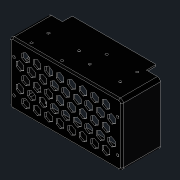
# Autodesk Inventor part: base45
Saved by Autodesk Inventor 2022 (Build 260153000, 153)
## iProperties
Created: 2021-08-30
Part Number: base45
Material: ABS プラスチック
Document SubType Name: Modeling
Designer: Yuta Kage
Density: 1.06 g/cm^3
Appearance: 滑らか - 黒
Author: Yuta Kage
Autodesk Inventor part; units mm, degrees
ref_plane "YZ Plane" through (0, 0, 0) normal (1, 0, 0) x (0, 1, 0)
ref_plane "XZ Plane" through (0, 0, 0) normal (0, 1, 0) x (-1, 0, 0)
ref_plane "XY Plane" through (0, 0, 0) normal (0, 0, 1) x (1, 0, 0)
sketch "スケッチ1" plane through (0, 0, 0) normal (0, 0, 1) x (1, 0, 0)
  line L0 (-70.25, -50) -> (70.25, -50) construction
  line L1 (70.25, -50) -> (70.25, 25) construction
  line L2 (70.25, 25) -> (-70.25, 25) construction
  line L3 (-70.25, 25) -> (-70.25, -50) construction
  line L4 (73.25, -53) -> (-73.25, -53)
  line L5 (-73.25, -53) -> (-73.25, 28)
  line L6 (-73.25, 28) -> (73.25, 28)
  line L7 (73.25, 28) -> (73.25, -53)
  point P0 (0, 0)
  dimension "d0" = 140.5
  dimension "d2" = 3
  dimension "d3" = 3
  dimension "d25" = 25
  dimension "d26" = 50
  dimension "d27" = 3
  dimension "d28" = 70.25
  dimension "d29" = 3
  constraints: 16 end point, 4 parallel, 2 horizontal, 2 perpendicular
  measures "d0" distance of L2.end L1.end
  measures "d2" distance between parallel lines of L6 L2
  measures "d3" distance between parallel lines of L5 L3
  measures "d25" distance from line of L2 point (0, 0)
  measures "d26" distance from line of L0 point (0, 0)
  measures "d27" distance between parallel lines of L1 L7
  measures "d28" distance from line of point (0, 0) L1
  measures "d29" distance between parallel lines of L0 L4
extrude "押し出し1" add sketch "スケッチ1" along normal blind 52.42
fillet "フィレット1" radius 4 4 edges at (73.25, 28, 26.21) (-73.25, 28, 26.21) (73.25, -53, 26.21) (-73.25, -53, 26.21)
fillet "フィレット2" radius 2 8 edges at (0, 28, 52.42) (-72.0784, 26.8284, 52.42) (-73.25, -12.5, 52.42) (-72.0784, -51.8284, 52.42) (0, -53, 52.42) (72.0784, -51.8284, 52.42) (73.25, -12.5, 52.42) (72.0784, 26.8284, 52.42)
shell "シェル1" thickness 2 removed faces 0
sketch "スケッチ2" plane through (0, 0, 0) normal (0, 0, -1) x (-1, 0, 0)
  arc A0 (69.25, -53) -> (73.25, -49) centre (69.25, -49) ccw projected
  line L0 (73.25, 24) -> (73.25, -49) projected
  arc A1 (73.25, 24) -> (69.25, 28) centre (69.25, 24) ccw projected
  line L1 (-69.25, 28) -> (69.25, 28) projected
  arc A2 (-69.25, 28) -> (-73.25, 24) centre (-69.25, 24) ccw projected
  line L2 (-73.25, -49) -> (-73.25, 24) projected
  arc A3 (-73.25, -49) -> (-69.25, -53) centre (-69.25, -49) ccw projected
  line L3 (69.25, -53) -> (-69.25, -53) projected
  point P0 (0, 0)
extrude "押し出し2" cut sketch "スケッチ2" against normal blind 2
sketch "スケッチ4" plane through (-69.25, -53, 50.42) normal (0, -1, 0) x (1, 0, 0)
  line L0 (138.5, -48.42) -> (0, -48.42) projected
  line L1 (124.25, -23.42) -> (14.25, -23.42)
  line L2 (14.25, -23.42) -> (14.25, -48.42)
  line L3 (14.25, -48.42) -> (124.25, -48.42)
  line L4 (124.25, -48.42) -> (124.25, -23.42)
  line L5 (124.25, -23.42) -> (14.25, -48.42) construction
  line L6 (14.25, -23.42) -> (124.25, -48.42) construction
  point P0 (69.25, -50.42)
  point P1 (69.25, -35.92)
  point P2 (69.25, -35.92)
  point P3 (124.25, -48.42)
  dimension "d21" = 110
  dimension "d22" = 25
  constraints: 12 end point, 3 midpoint, 2 parallel, 1 horizontal, 1 perpendicular, 1 point on line, 1 vertical alignment
  measures "d21" distance of L1.start L1.end
  measures "d22" distance of L3.end L1.start
extrude "押し出し3" cut sketch "スケッチ4" against normal blind 5
fillet "フィレット3" radius 5 2 edges at (55, -52, 27) (-55, -52, 27)
sketch "スケッチ3" plane through (0, 0, 52.42) normal (0, 0, 1) x (1, 0, 0)
  line L0 (73.25, 28) -> (-73.25, 28) projected
  line L1 (-73.25, 28) -> (-73.25, -53) projected
  line L2 (-73.25, -53) -> (73.25, -53) projected
  line L3 (73.25, -53) -> (73.25, 28) projected
  line L4 (-67.75, -36.75) -> (67.75, -36.75)
  line L5 (67.75, -36.75) -> (67.75, 6.75)
  line L6 (67.75, 6.75) -> (-67.75, 6.75)
  line L7 (-67.75, 6.75) -> (-67.75, -36.75)
  line L8 (-67.75, -36.75) -> (67.75, 6.75) construction
  line L9 (67.75, -36.75) -> (-67.75, 6.75) construction
  point P0 (88.6427, 28.7758)
  point P1 (88.6427, -28.7758)
  point P2 (0, 0)
  point P3 (0, -15)
  dimension "d19" = 135.5
  dimension "d20" = 43.5
  dimension "d103" = 81
  dimension "d106" = 15
  constraints: 12 end point, 2 parallel, 1 horizontal, 1 midpoint, 1 perpendicular, 1 vertical alignment
  measures "d19" distance of L5.end L6.end
  measures "d20" distance of L6.end L4.start
  measures "d103" distance between parallel lines of L2 L0
  measures "d106" distance of point (0, -15) point (0, 0)
hole "穴1" at (88.6427, -28.7758, 52.42) at (88.6427, 28.7758, 52.42) at (-67.75, 6.75, 52.42) at (-67.75, -36.75, 52.42) at (67.75, 6.75, 52.42) at (67.75, -36.75, 52.42) direction (0, 0, -1) diameter 3.4 end through all clearance for "Socket Head Cap Screw" size "M3" standard "Ansi Metric M Profile"
sketch "スケッチ5" plane through (-73.25, -49, 50.42) normal (-1, 0, 0) x (0, 0, 1)
  line L0 (-13.92, 52) -> (-21.92, 52)
  line L1 (-21.92, 52) -> (-21.92, 40)
  line L2 (-21.92, 40) -> (-13.92, 40)
  line L3 (-13.92, 40) -> (-13.92, 52)
  line L4 (-13.92, 52) -> (-21.92, 40) construction
  line L5 (-21.92, 52) -> (-13.92, 40) construction
  line L6 (0, 77) -> (-48.42, 77) projected
  line L7 (-48.42, 73) -> (-48.42, 0) projected
  line L8 (-30.92, 52) -> (-38.92, 52)
  line L9 (-38.92, 52) -> (-38.92, 40)
  line L10 (-38.92, 40) -> (-30.92, 40)
  line L11 (-30.92, 40) -> (-30.92, 52)
  line L12 (-30.92, 52) -> (-38.92, 40) construction
  line L13 (-38.92, 52) -> (-30.92, 40) construction
  point P0 (-50.42, 49)
  point P1 (-17.92, 46)
  point P2 (-34.92, 46)
  dimension "d31" = 31
  dimension "d32" = 30.5
  dimension "d33" = 8
  dimension "d34" = 12
  dimension "d37" = 17
  constraints: 24 end point, 4 midpoint, 2 horizontal, 2 parallel, 1 collinear, 1 perpendicular, 10 other
  measures "d31" distance from line of L6 point (-17.92, 46)
  measures "d32" distance from line of L7 point (-17.92, 46)
  measures "d33" distance of L1.end L2.end
  measures "d34" distance of L2.end L0.start
  measures "d37" distance of L0.start L8.start
extrude "押し出し4" cut sketch "スケッチ5" against normal blind 10
fillet "フィレット4" radius 1 8 edges at (-72.25, -9, 19.5) (-72.25, -9, 11.5) (-72.25, 3, 11.5) (-72.25, 3, 19.5) (-72.25, -9, 36.5) (-72.25, -9, 28.5) (-72.25, 3, 28.5) (-72.25, 3, 36.5)
sketch "スケッチ6" plane through (0, 0, 2) normal (0, 0, -1) x (-1, 0, 0)
  line L0 (69.25, 26) -> (-69.25, 26) projected
  line L1 (-69.25, 28) -> (69.25, 28) projected
  line L2 (55, 26) -> (-55, 26)
  line L3 (-55, 26) -> (-55, 28)
  line L4 (-55, 28) -> (55, 28)
  line L5 (55, 28) -> (55, 26)
  point P0 (0, 0)
  dimension "d45" = 55
  dimension "d46" = 55
  constraints: 8 end point, 2 parallel, 2 point on line, 1 horizontal, 1 perpendicular
  measures "d45" distance from line of point (0, 0) L3
  measures "d46" distance from line of L5 point (0, 0)
extrude "押し出し5" add sketch "スケッチ6" along normal blind 13
sketch "スケッチ7" plane through (0, 0, 52.42) normal (0, 0, 1) x (1, 0, 0)
  line L0 (-102.55, 0) -> (102.55, 0) construction
  line L1 (0, -69.2) -> (0, 44.2) projected
  line L2 (-69.25, -53) -> (69.25, -53) construction
  line L3 (69.25, 28) -> (-69.25, 28) projected
  line L4 (-60, -57.2446) -> (-65, -54.3579) construction
  line L5 (-65, -54.3579) -> (-65, -48.5844) construction
  line L6 (-65, -48.5844) -> (-60, -45.6976) construction
  line L7 (-60, -45.6976) -> (-55, -48.5844) construction
  line L8 (-55, -48.5844) -> (-55, -54.3579) construction
  line L9 (-55, -54.3579) -> (-60, -57.2446) construction
  line L10 (-67.5, -44.2543) -> (-72.5, -41.3675) construction
  line L11 (-72.5, -41.3675) -> (-72.5, -35.594) construction
  line L12 (-72.5, -35.594) -> (-67.5, -32.7073) construction
  line L13 (-67.5, -32.7073) -> (-62.5, -35.594) construction
  line L14 (-62.5, -35.594) -> (-62.5, -41.3675) construction
  line L15 (-62.5, -41.3675) -> (-67.5, -44.2543) construction
  line L16 (-60, -51.4711) -> (-67.5, -38.4808) construction
  line L17 (-57.5, -41.3675) -> (-57.5, -35.594)
  line L18 (-52.5, -44.2543) -> (-57.5, -41.3675)
  line L19 (-57.5, -35.594) -> (-52.5, -32.7073)
  line L20 (-47.5, -41.3675) -> (-52.5, -44.2543)
  line L21 (-52.5, -32.7073) -> (-47.5, -35.594)
  line L22 (-47.5, -35.594) -> (-47.5, -41.3675)
  line L23 (-50, -54.3579) -> (-50, -48.5844) construction
  line L24 (-45, -57.2446) -> (-50, -54.3579) construction
  line L25 (-50, -48.5844) -> (-45, -45.6976) construction
  line L26 (-45, -51.4711) -> (-52.5, -38.4808) construction
  line L27 (-40, -54.3579) -> (-45, -57.2446) construction
  line L28 (-40, -48.5844) -> (-40, -54.3579) construction
  line L29 (-45, -45.6976) -> (-40, -48.5844) construction
  line L30 (-72.5, -15.3868) -> (-72.5, -9.6132) construction
  line L31 (-67.5, -18.2735) -> (-72.5, -15.3868) construction
  line L32 (-72.5, -9.6132) -> (-67.5, -6.7265) construction
  line L33 (-62.5, -15.3868) -> (-67.5, -18.2735) construction
  line L34 (-67.5, -6.7265) -> (-62.5, -9.6132) construction
  line L35 (-62.5, -9.6132) -> (-62.5, -15.3868) construction
  line L36 (-65, -28.3771) -> (-65, -22.6036)
  line L37 (-60, -31.2639) -> (-65, -28.3771)
  line L38 (-65, -22.6036) -> (-60, -19.7169)
  line L39 (-60, -25.4904) -> (-67.5, -12.5) construction
  line L40 (-55, -28.3771) -> (-60, -31.2639)
  line L41 (-55, -22.6036) -> (-55, -28.3771)
  line L42 (-60, -19.7169) -> (-55, -22.6036)
  line L43 (-57.5, -15.3868) -> (-57.5, -9.6132)
  line L44 (-52.5, -18.2735) -> (-57.5, -15.3868)
  line L45 (-57.5, -9.6132) -> (-52.5, -6.7265)
  line L46 (-47.5, -15.3868) -> (-52.5, -18.2735)
  line L47 (-52.5, -6.7265) -> (-47.5, -9.6132)
  line L48 (-47.5, -9.6132) -> (-47.5, -15.3868)
  line L49 (-50, -28.3771) -> (-50, -22.6036)
  line L50 (-45, -31.2639) -> (-50, -28.3771)
  line L51 (-50, -22.6036) -> (-45, -19.7169)
  line L52 (-45, -25.4904) -> (-52.5, -12.5) construction
  line L53 (-40, -28.3771) -> (-45, -31.2639)
  line L54 (-40, -22.6036) -> (-40, -28.3771)
  line L55 (-45, -19.7169) -> (-40, -22.6036)
  line L56 (-42.5, -41.3675) -> (-42.5, -35.594)
  line L57 (-37.5, -44.2543) -> (-42.5, -41.3675)
  line L58 (-42.5, -35.594) -> (-37.5, -32.7073)
  line L59 (-32.5, -41.3675) -> (-37.5, -44.2543)
  line L60 (-37.5, -32.7073) -> (-32.5, -35.594)
  line L61 (-32.5, -35.594) -> (-32.5, -41.3675)
  line L62 (-35, -54.3579) -> (-35, -48.5844) construction
  line L63 (-30, -57.2446) -> (-35, -54.3579) construction
  line L64 (-35, -48.5844) -> (-30, -45.6976) construction
  line L65 (-30, -51.4711) -> (-37.5, -38.4808) construction
  line L66 (-25, -54.3579) -> (-30, -57.2446) construction
  line L67 (-25, -48.5844) -> (-25, -54.3579) construction
  line L68 (-30, -45.6976) -> (-25, -48.5844) construction
  line L69 (-42.5, -15.3868) -> (-42.5, -9.6132)
  line L70 (-37.5, -18.2735) -> (-42.5, -15.3868)
  line L71 (-42.5, -9.6132) -> (-37.5, -6.7265)
  line L72 (-32.5, -15.3868) -> (-37.5, -18.2735)
  line L73 (-37.5, -6.7265) -> (-32.5, -9.6132)
  line L74 (-32.5, -9.6132) -> (-32.5, -15.3868)
  line L75 (-35, -28.3771) -> (-35, -22.6036)
  line L76 (-30, -31.2639) -> (-35, -28.3771)
  line L77 (-35, -22.6036) -> (-30, -19.7169)
  line L78 (-30, -25.4904) -> (-37.5, -12.5) construction
  line L79 (-25, -28.3771) -> (-30, -31.2639)
  line L80 (-25, -22.6036) -> (-25, -28.3771)
  line L81 (-30, -19.7169) -> (-25, -22.6036)
  line L82 (-27.5, -41.3675) -> (-27.5, -35.594)
  line L83 (-22.5, -44.2543) -> (-27.5, -41.3675)
  line L84 (-27.5, -35.594) -> (-22.5, -32.7073)
  line L85 (-17.5, -41.3675) -> (-22.5, -44.2543)
  line L86 (-22.5, -32.7073) -> (-17.5, -35.594)
  line L87 (-17.5, -35.594) -> (-17.5, -41.3675)
  line L88 (-20, -54.3579) -> (-20, -48.5844) construction
  line L89 (-15, -57.2446) -> (-20, -54.3579) construction
  line L90 (-20, -48.5844) -> (-15, -45.6976) construction
  line L91 (-15, -51.4711) -> (-22.5, -38.4808) construction
  line L92 (-10, -54.3579) -> (-15, -57.2446) construction
  line L93 (-10, -48.5844) -> (-10, -54.3579) construction
  line L94 (-15, -45.6976) -> (-10, -48.5844) construction
  line L95 (-27.5, -15.3868) -> (-27.5, -9.6132)
  line L96 (-22.5, -18.2735) -> (-27.5, -15.3868)
  line L97 (-27.5, -9.6132) -> (-22.5, -6.7265)
  line L98 (-17.5, -15.3868) -> (-22.5, -18.2735)
  line L99 (-22.5, -6.7265) -> (-17.5, -9.6132)
  line L100 (-17.5, -9.6132) -> (-17.5, -15.3868)
  line L101 (-20, -28.3771) -> (-20, -22.6036)
  line L102 (-15, -31.2639) -> (-20, -28.3771)
  line L103 (-20, -22.6036) -> (-15, -19.7169)
  line L104 (-15, -25.4904) -> (-22.5, -12.5) construction
  line L105 (-10, -28.3771) -> (-15, -31.2639)
  line L106 (-10, -22.6036) -> (-10, -28.3771)
  line L107 (-15, -19.7169) -> (-10, -22.6036)
  line L108 (-12.5, -41.3675) -> (-12.5, -35.594)
  line L109 (-7.5, -44.2543) -> (-12.5, -41.3675)
  line L110 (-12.5, -35.594) -> (-7.5, -32.7073)
  line L111 (-2.5, -41.3675) -> (-7.5, -44.2543)
  line L112 (-7.5, -32.7073) -> (-2.5, -35.594)
  line L113 (-2.5, -35.594) -> (-2.5, -41.3675)
  line L114 (-5, -54.3579) -> (-5, -48.5844) construction
  line L115 (0, -57.2446) -> (-5, -54.3579) construction
  line L116 (-5, -48.5844) -> (0, -45.6976) construction
  line L117 (0, -51.4711) -> (-7.5, -38.4808) construction
  line L118 (5, -54.3579) -> (0, -57.2446) construction
  line L119 (5, -48.5844) -> (5, -54.3579) construction
  line L120 (0, -45.6976) -> (5, -48.5844) construction
  line L121 (-12.5, -15.3868) -> (-12.5, -9.6132)
  line L122 (-7.5, -18.2735) -> (-12.5, -15.3868)
  line L123 (-12.5, -9.6132) -> (-7.5, -6.7265)
  line L124 (-2.5, -15.3868) -> (-7.5, -18.2735)
  line L125 (-7.5, -6.7265) -> (-2.5, -9.6132)
  line L126 (-2.5, -9.6132) -> (-2.5, -15.3868)
  line L127 (-5, -28.3771) -> (-5, -22.6036)
  line L128 (0, -31.2639) -> (-5, -28.3771)
  line L129 (-5, -22.6036) -> (0, -19.7169)
  line L130 (0, -25.4904) -> (-7.5, -12.5) construction
  line L131 (5, -28.3771) -> (0, -31.2639)
  line L132 (5, -22.6036) -> (5, -28.3771)
  line L133 (0, -19.7169) -> (5, -22.6036)
  line L134 (2.5, -41.3675) -> (2.5, -35.594)
  line L135 (7.5, -44.2543) -> (2.5, -41.3675)
  line L136 (2.5, -35.594) -> (7.5, -32.7073)
  line L137 (12.5, -41.3675) -> (7.5, -44.2543)
  line L138 (7.5, -32.7073) -> (12.5, -35.594)
  line L139 (12.5, -35.594) -> (12.5, -41.3675)
  line L140 (10, -54.3579) -> (10, -48.5844) construction
  line L141 (15, -57.2446) -> (10, -54.3579) construction
  line L142 (10, -48.5844) -> (15, -45.6976) construction
  line L143 (15, -51.4711) -> (7.5, -38.4808) construction
  line L144 (20, -54.3579) -> (15, -57.2446) construction
  line L145 (20, -48.5844) -> (20, -54.3579) construction
  line L146 (15, -45.6976) -> (20, -48.5844) construction
  line L147 (2.5, -15.3868) -> (2.5, -9.6132)
  line L148 (7.5, -18.2735) -> (2.5, -15.3868)
  line L149 (2.5, -9.6132) -> (7.5, -6.7265)
  line L150 (12.5, -15.3868) -> (7.5, -18.2735)
  line L151 (7.5, -6.7265) -> (12.5, -9.6132)
  line L152 (12.5, -9.6132) -> (12.5, -15.3868)
  line L153 (10, -28.3771) -> (10, -22.6036)
  line L154 (15, -31.2639) -> (10, -28.3771)
  line L155 (10, -22.6036) -> (15, -19.7169)
  line L156 (15, -25.4904) -> (7.5, -12.5) construction
  line L157 (20, -28.3771) -> (15, -31.2639)
  line L158 (20, -22.6036) -> (20, -28.3771)
  line L159 (15, -19.7169) -> (20, -22.6036)
  line L160 (17.5, -41.3675) -> (17.5, -35.594)
  line L161 (22.5, -44.2543) -> (17.5, -41.3675)
  line L162 (17.5, -35.594) -> (22.5, -32.7073)
  line L163 (27.5, -41.3675) -> (22.5, -44.2543)
  line L164 (22.5, -32.7073) -> (27.5, -35.594)
  line L165 (27.5, -35.594) -> (27.5, -41.3675)
  line L166 (25, -54.3579) -> (25, -48.5844) construction
  line L167 (30, -57.2446) -> (25, -54.3579) construction
  line L168 (25, -48.5844) -> (30, -45.6976) construction
  line L169 (30, -51.4711) -> (22.5, -38.4808) construction
  line L170 (35, -54.3579) -> (30, -57.2446) construction
  line L171 (35, -48.5844) -> (35, -54.3579) construction
  line L172 (30, -45.6976) -> (35, -48.5844) construction
  line L173 (17.5, -15.3868) -> (17.5, -9.6132)
  line L174 (22.5, -18.2735) -> (17.5, -15.3868)
  line L175 (17.5, -9.6132) -> (22.5, -6.7265)
  line L176 (27.5, -15.3868) -> (22.5, -18.2735)
  line L177 (22.5, -6.7265) -> (27.5, -9.6132)
  line L178 (27.5, -9.6132) -> (27.5, -15.3868)
  line L179 (25, -28.3771) -> (25, -22.6036)
  line L180 (30, -31.2639) -> (25, -28.3771)
  line L181 (25, -22.6036) -> (30, -19.7169)
  line L182 (30, -25.4904) -> (22.5, -12.5) construction
  line L183 (35, -28.3771) -> (30, -31.2639)
  line L184 (35, -22.6036) -> (35, -28.3771)
  line L185 (30, -19.7169) -> (35, -22.6036)
  line L186 (32.5, -41.3675) -> (32.5, -35.594)
  line L187 (37.5, -44.2543) -> (32.5, -41.3675)
  line L188 (32.5, -35.594) -> (37.5, -32.7073)
  line L189 (42.5, -41.3675) -> (37.5, -44.2543)
  line L190 (37.5, -32.7073) -> (42.5, -35.594)
  line L191 (42.5, -35.594) -> (42.5, -41.3675)
  line L192 (40, -54.3579) -> (40, -48.5844) construction
  line L193 (45, -57.2446) -> (40, -54.3579) construction
  line L194 (40, -48.5844) -> (45, -45.6976) construction
  line L195 (45, -51.4711) -> (37.5, -38.4808) construction
  line L196 (50, -54.3579) -> (45, -57.2446) construction
  line L197 (50, -48.5844) -> (50, -54.3579) construction
  line L198 (45, -45.6976) -> (50, -48.5844) construction
  line L199 (32.5, -15.3868) -> (32.5, -9.6132)
  line L200 (37.5, -18.2735) -> (32.5, -15.3868)
  line L201 (32.5, -9.6132) -> (37.5, -6.7265)
  line L202 (42.5, -15.3868) -> (37.5, -18.2735)
  line L203 (37.5, -6.7265) -> (42.5, -9.6132)
  line L204 (42.5, -9.6132) -> (42.5, -15.3868)
  line L205 (40, -28.3771) -> (40, -22.6036)
  line L206 (45, -31.2639) -> (40, -28.3771)
  line L207 (40, -22.6036) -> (45, -19.7169)
  line L208 (45, -25.4904) -> (37.5, -12.5) construction
  line L209 (50, -28.3771) -> (45, -31.2639)
  line L210 (50, -22.6036) -> (50, -28.3771)
  line L211 (45, -19.7169) -> (50, -22.6036)
  line L212 (47.5, -41.3675) -> (47.5, -35.594)
  line L213 (52.5, -44.2543) -> (47.5, -41.3675)
  line L214 (47.5, -35.594) -> (52.5, -32.7073)
  line L215 (57.5, -41.3675) -> (52.5, -44.2543)
  line L216 (52.5, -32.7073) -> (57.5, -35.594)
  line L217 (57.5, -35.594) -> (57.5, -41.3675)
  line L218 (55, -54.3579) -> (55, -48.5844) construction
  line L219 (60, -57.2446) -> (55, -54.3579) construction
  line L220 (55, -48.5844) -> (60, -45.6976) construction
  line L221 (60, -51.4711) -> (52.5, -38.4808) construction
  line L222 (65, -54.3579) -> (60, -57.2446) construction
  line L223 (65, -48.5844) -> (65, -54.3579) construction
  line L224 (60, -45.6976) -> (65, -48.5844) construction
  line L225 (47.5, -15.3868) -> (47.5, -9.6132)
  line L226 (52.5, -18.2735) -> (47.5, -15.3868)
  line L227 (47.5, -9.6132) -> (52.5, -6.7265)
  line L228 (57.5, -15.3868) -> (52.5, -18.2735)
  line L229 (52.5, -6.7265) -> (57.5, -9.6132)
  line L230 (57.5, -9.6132) -> (57.5, -15.3868)
  line L231 (55, -28.3771) -> (55, -22.6036)
  line L232 (60, -31.2639) -> (55, -28.3771)
  line L233 (55, -22.6036) -> (60, -19.7169)
  line L234 (60, -25.4904) -> (52.5, -12.5) construction
  line L235 (65, -28.3771) -> (60, -31.2639)
  line L236 (65, -22.6036) -> (65, -28.3771)
  line L237 (60, -19.7169) -> (65, -22.6036)
  line L238 (62.5, -41.3675) -> (62.5, -35.594) construction
  line L239 (67.5, -44.2543) -> (62.5, -41.3675) construction
  line L240 (62.5, -35.594) -> (67.5, -32.7073) construction
  line L241 (72.5, -41.3675) -> (67.5, -44.2543) construction
  line L242 (67.5, -32.7073) -> (72.5, -35.594) construction
  line L243 (72.5, -35.594) -> (72.5, -41.3675) construction
  line L244 (70, -54.3579) -> (70, -48.5844) construction
  line L245 (75, -57.2446) -> (70, -54.3579) construction
  line L246 (70, -48.5844) -> (75, -45.6976) construction
  line L247 (75, -51.4711) -> (67.5, -38.4808) construction
  line L248 (80, -54.3579) -> (75, -57.2446) construction
  line L249 (80, -48.5844) -> (80, -54.3579) construction
  line L250 (75, -45.6976) -> (80, -48.5844) construction
  line L251 (62.5, -15.3868) -> (62.5, -9.6132) construction
  line L252 (67.5, -18.2735) -> (62.5, -15.3868) construction
  line L253 (62.5, -9.6132) -> (67.5, -6.7265) construction
  line L254 (72.5, -15.3868) -> (67.5, -18.2735) construction
  line L255 (67.5, -6.7265) -> (72.5, -9.6132) construction
  line L256 (72.5, -9.6132) -> (72.5, -15.3868) construction
  line L257 (70, -28.3771) -> (70, -22.6036) construction
  line L258 (75, -31.2639) -> (70, -28.3771) construction
  line L259 (70, -22.6036) -> (75, -19.7169) construction
  line L260 (75, -25.4904) -> (67.5, -12.5) construction
  line L261 (80, -28.3771) -> (75, -31.2639) construction
  line L262 (80, -22.6036) -> (80, -28.3771) construction
  line L263 (75, -19.7169) -> (80, -22.6036) construction
  line L264 (-72.5, 10.594) -> (-72.5, 16.3675)
  line L265 (-67.5, 7.7073) -> (-72.5, 10.594)
  line L266 (-72.5, 16.3675) -> (-67.5, 19.2543)
  line L267 (-62.5, 10.594) -> (-67.5, 7.7073)
  line L268 (-67.5, 19.2543) -> (-62.5, 16.3675)
  line L269 (-62.5, 16.3675) -> (-62.5, 10.594)
  line L270 (-65, -2.3964) -> (-65, 3.3771)
  line L271 (-60, -5.2831) -> (-65, -2.3964)
  line L272 (-65, 3.3771) -> (-60, 6.2639)
  line L273 (-60, 0.4904) -> (-67.5, 13.4808) construction
  line L274 (-55, -2.3964) -> (-60, -5.2831)
  line L275 (-55, 3.3771) -> (-55, -2.3964)
  line L276 (-60, 6.2639) -> (-55, 3.3771)
  line L277 (-57.5, 10.594) -> (-57.5, 16.3675)
  line L278 (-52.5, 7.7073) -> (-57.5, 10.594)
  line L279 (-57.5, 16.3675) -> (-52.5, 19.2543)
  line L280 (-47.5, 10.594) -> (-52.5, 7.7073)
  line L281 (-52.5, 19.2543) -> (-47.5, 16.3675)
  line L282 (-47.5, 16.3675) -> (-47.5, 10.594)
  line L283 (-50, -2.3964) -> (-50, 3.3771)
  line L284 (-45, -5.2831) -> (-50, -2.3964)
  line L285 (-50, 3.3771) -> (-45, 6.2639)
  line L286 (-45, 0.4904) -> (-52.5, 13.4808) construction
  line L287 (-40, -2.3964) -> (-45, -5.2831)
  line L288 (-40, 3.3771) -> (-40, -2.3964)
  line L289 (-45, 6.2639) -> (-40, 3.3771)
  line L290 (-42.5, 10.594) -> (-42.5, 16.3675)
  line L291 (-37.5, 7.7073) -> (-42.5, 10.594)
  line L292 (-42.5, 16.3675) -> (-37.5, 19.2543)
  line L293 (-32.5, 10.594) -> (-37.5, 7.7073)
  line L294 (-37.5, 19.2543) -> (-32.5, 16.3675)
  line L295 (-32.5, 16.3675) -> (-32.5, 10.594)
  line L296 (-35, -2.3964) -> (-35, 3.3771)
  line L297 (-30, -5.2831) -> (-35, -2.3964)
  line L298 (-35, 3.3771) -> (-30, 6.2639)
  line L299 (-30, 0.4904) -> (-37.5, 13.4808) construction
  line L300 (-25, -2.3964) -> (-30, -5.2831)
  line L301 (-25, 3.3771) -> (-25, -2.3964)
  line L302 (-30, 6.2639) -> (-25, 3.3771)
  line L303 (-27.5, 10.594) -> (-27.5, 16.3675)
  line L304 (-22.5, 7.7073) -> (-27.5, 10.594)
  line L305 (-27.5, 16.3675) -> (-22.5, 19.2543)
  line L306 (-17.5, 10.594) -> (-22.5, 7.7073)
  line L307 (-22.5, 19.2543) -> (-17.5, 16.3675)
  line L308 (-17.5, 16.3675) -> (-17.5, 10.594)
  line L309 (-20, -2.3964) -> (-20, 3.3771)
  line L310 (-15, -5.2831) -> (-20, -2.3964)
  line L311 (-20, 3.3771) -> (-15, 6.2639)
  line L312 (-15, 0.4904) -> (-22.5, 13.4808) construction
  line L313 (-10, -2.3964) -> (-15, -5.2831)
  line L314 (-10, 3.3771) -> (-10, -2.3964)
  line L315 (-15, 6.2639) -> (-10, 3.3771)
  line L316 (-12.5, 10.594) -> (-12.5, 16.3675)
  line L317 (-7.5, 7.7073) -> (-12.5, 10.594)
  line L318 (-12.5, 16.3675) -> (-7.5, 19.2543)
  line L319 (-2.5, 10.594) -> (-7.5, 7.7073)
  line L320 (-7.5, 19.2543) -> (-2.5, 16.3675)
  line L321 (-2.5, 16.3675) -> (-2.5, 10.594)
  line L322 (-5, -2.3964) -> (-5, 3.3771)
  line L323 (0, -5.2831) -> (-5, -2.3964)
  line L324 (-5, 3.3771) -> (0, 6.2639)
  line L325 (0, 0.4904) -> (-7.5, 13.4808) construction
  line L326 (5, -2.3964) -> (0, -5.2831)
  line L327 (5, 3.3771) -> (5, -2.3964)
  line L328 (0, 6.2639) -> (5, 3.3771)
  line L329 (2.5, 10.594) -> (2.5, 16.3675)
  line L330 (7.5, 7.7073) -> (2.5, 10.594)
  line L331 (2.5, 16.3675) -> (7.5, 19.2543)
  line L332 (12.5, 10.594) -> (7.5, 7.7073)
  line L333 (7.5, 19.2543) -> (12.5, 16.3675)
  line L334 (12.5, 16.3675) -> (12.5, 10.594)
  line L335 (10, -2.3964) -> (10, 3.3771)
  line L336 (15, -5.2831) -> (10, -2.3964)
  line L337 (10, 3.3771) -> (15, 6.2639)
  line L338 (15, 0.4904) -> (7.5, 13.4808) construction
  line L339 (20, -2.3964) -> (15, -5.2831)
  line L340 (20, 3.3771) -> (20, -2.3964)
  line L341 (15, 6.2639) -> (20, 3.3771)
  line L342 (17.5, 10.594) -> (17.5, 16.3675)
  line L343 (22.5, 7.7073) -> (17.5, 10.594)
  line L344 (17.5, 16.3675) -> (22.5, 19.2543)
  line L345 (27.5, 10.594) -> (22.5, 7.7073)
  line L346 (22.5, 19.2543) -> (27.5, 16.3675)
  line L347 (27.5, 16.3675) -> (27.5, 10.594)
  line L348 (25, -2.3964) -> (25, 3.3771)
  line L349 (30, -5.2831) -> (25, -2.3964)
  line L350 (25, 3.3771) -> (30, 6.2639)
  line L351 (30, 0.4904) -> (22.5, 13.4808) construction
  line L352 (35, -2.3964) -> (30, -5.2831)
  line L353 (35, 3.3771) -> (35, -2.3964)
  line L354 (30, 6.2639) -> (35, 3.3771)
  line L355 (32.5, 10.594) -> (32.5, 16.3675)
  line L356 (37.5, 7.7073) -> (32.5, 10.594)
  line L357 (32.5, 16.3675) -> (37.5, 19.2543)
  line L358 (42.5, 10.594) -> (37.5, 7.7073)
  line L359 (37.5, 19.2543) -> (42.5, 16.3675)
  line L360 (42.5, 16.3675) -> (42.5, 10.594)
  line L361 (40, -2.3964) -> (40, 3.3771)
  line L362 (45, -5.2831) -> (40, -2.3964)
  line L363 (40, 3.3771) -> (45, 6.2639)
  line L364 (45, 0.4904) -> (37.5, 13.4808) construction
  line L365 (50, -2.3964) -> (45, -5.2831)
  line L366 (50, 3.3771) -> (50, -2.3964)
  line L367 (45, 6.2639) -> (50, 3.3771)
  line L368 (47.5, 10.594) -> (47.5, 16.3675)
  line L369 (52.5, 7.7073) -> (47.5, 10.594)
  line L370 (47.5, 16.3675) -> (52.5, 19.2543)
  line L371 (57.5, 10.594) -> (52.5, 7.7073)
  line L372 (52.5, 19.2543) -> (57.5, 16.3675)
  line L373 (57.5, 16.3675) -> (57.5, 10.594)
  line L374 (55, -2.3964) -> (55, 3.3771)
  line L375 (60, -5.2831) -> (55, -2.3964)
  line L376 (55, 3.3771) -> (60, 6.2639)
  line L377 (60, 0.4904) -> (52.5, 13.4808) construction
  line L378 (65, -2.3964) -> (60, -5.2831)
  line L379 (65, 3.3771) -> (65, -2.3964)
  line L380 (60, 6.2639) -> (65, 3.3771)
  line L381 (62.5, 10.594) -> (62.5, 16.3675)
  line L382 (67.5, 7.7073) -> (62.5, 10.594)
  line L383 (62.5, 16.3675) -> (67.5, 19.2543)
  line L384 (72.5, 10.594) -> (67.5, 7.7073)
  line L385 (67.5, 19.2543) -> (72.5, 16.3675)
  line L386 (72.5, 16.3675) -> (72.5, 10.594)
  line L387 (70, -2.3964) -> (70, 3.3771) construction
  line L388 (75, -5.2831) -> (70, -2.3964) construction
  line L389 (70, 3.3771) -> (75, 6.2639) construction
  line L390 (75, 0.4904) -> (67.5, 13.4808) construction
  line L391 (80, -2.3964) -> (75, -5.2831) construction
  line L392 (80, 3.3771) -> (80, -2.3964) construction
  line L393 (75, 6.2639) -> (80, 3.3771) construction
  point P0 (0, -11.9304)
  dimension "d82" = 81
  dimension "d85" = 10
  dimension "d86" = 10
  dimension "d87" = 5
  dimension "d92" = 15
  dimension "d95" = 25.9808
  dimension "d98" = 12.9904
  dimension "d99" = 5
  dimension "d100" = 0
  dimension "d105" = 40.5
  constraints: 780 end point, 3 vertical alignment, 1 horizontal, 1 vertical, 810 other
  measures "d82" distance between parallel lines of L2 L3
  measures "d85" distance between parallel lines of L5 L8
  measures "d86" distance between parallel lines of L11 L14
  measures "d87" distance between parallel lines of L6 L15
  measures "d92" distance of L11.end L17.end
  measures "d95" distance of L11.end L30.end
  measures "d98" vertical distance of L16.end L16.start
  measures "d99" distance between parallel lines of L18 L7
  measures "d100" distance from line of L1 L117.start
  measures "d105" distance from line of L2 L156.end
extrude "押し出し6" cut sketch "スケッチ7" against normal blind 10 contours L128 L127 L129 L1 | L1 L133 L132 L131 | L323 L322 L324 L1 | L1 L328 L327 L326 | L17 L19 L21 L22 L20 L18 | L36 L38 L42 L41 L40 L37 | L43 L45 L47 L48 L46 L44 | L49 L51 L55 L54 L53 L50 | L56 L58 L60 L61 L59 L57 | L69 L71 L73 L74 L72 L70 | L75 L77 L81 L80 L79 L76 | L82 L84 L86 L87 L85 L83 | L95 L97 L99 L100 L98 L96 | L101 L103 L107 L106 L105 L102 | L108 L110 L112 L113 L111 L109 | L121 L123 L125 L126 L124 L122 | L134 L136 L138 L139 L137 L135 | L147 L149 L151 L152 L150 L148 | L153 L155 L159 L158 L157 L154 | L160 L162 L164 L165 L163 L161 | L173 L175 L177 L178 L176 L174 | L179 L181 L185 L184 L183 L180 | L186 L188 L190 L191 L189 L187 | L199 L201 L203 L204 L202 L200 | L205 L207 L211 L210 L209 L206 | L212 L214 L216 L217 L215 L213 | L225 L227 L229 L230 L228 L226 | L231 L233 L237 L236 L235 L232 | L270 L272 L276 L275 L274 L271 | L277 L279 L281 L282 L280 L278 | L283 L285 L289 L288 L287 L284 | L290 L292 L294 L295 L293 L291 | L296 L298 L302 L301 L300 L297 | L303 L305 L307 L308 L306 L304 | L309 L311 L315 L314 L313 L310 | L316 L318 L320 L321 L319 L317 | L329 L331 L333 L334 L332 L330 | L335 L337 L341 L340 L339 L336 | L342 L344 L346 L347 L345 L343 | L348 L350 L354 L353 L352 L349 | L355 L357 L359 L360 L358 L356 | L361 L363 L367 L366 L365 L362 | L368 L370 L372 L373 L371 L369 | L374 L376 L380 L379 L378 L375
sketch "スケッチ8" plane through (-69.25, 28, 50.42) normal (0, 1, 0) x (1, 0, 0)
  line L0 (18.25, 4.17) -> (58.25, 4.17)
  line L1 (58.25, 4.17) -> (58.25, 26.42)
  line L2 (58.25, 26.42) -> (18.25, 26.42)
  line L3 (18.25, 26.42) -> (18.25, 4.17)
  line L4 (80.25, 18.17) -> (120.25, 18.17)
  line L5 (120.25, 18.17) -> (120.25, 40.42)
  line L6 (120.25, 40.42) -> (80.25, 40.42)
  line L7 (80.25, 40.42) -> (80.25, 18.17)
  point P0 (69.25, 50.42)
  dimension "d107" = 40
  dimension "d108" = 40
  dimension "d109" = 22.25
  dimension "d110" = 22.25
  dimension "d111" = 11
  dimension "d112" = 11
  dimension "d113" = 10
  dimension "d114" = 14
  constraints: 16 end point, 4 parallel, 2 horizontal, 2 perpendicular
  measures "d107" distance of L5.end L6.end
  measures "d108" distance of L1.end L2.end
  measures "d109" distance of L0.end L1.end
  measures "d110" distance of L6.end L4.start
  measures "d111" distance from line of point (69.25, 50.42) L7
  measures "d112" distance from line of point (69.25, 50.42) L1
  measures "d113" distance from line of L6 point (69.25, 50.42)
  measures "d114" distance between parallel lines of L6 L2
hole "穴2" at (11, 28, 10) at (51, 28, 32.25) at (-51, 28, 24) at (-11, 28, 46.25) at (11, 28, 32.25) at (-11, 28, 24) at (-51, 28, 46.25) at (51, 28, 10) direction (0, -1, 0) diameter 3.2 depth 8 tip angle 118 clearance for "Flat Head Machine Screw" size "M3" standard "Ansi Metric M Profile"
sketch "スケッチ9" plane through (-69.25, 28, 50.42) normal (0, 1, 0) x (1, 0, 0)
  line L0 (14.25, 48.42) -> (14.25, 61.42) projected
  line L1 (14.25, 61.42) -> (124.25, 61.42) projected
  line L2 (124.25, 48.42) -> (124.25, 61.42) projected
  line L3 (124.05, 48.42) -> (124.05, 61.22)
  line L4 (124.05, 61.22) -> (14.45, 61.22)
  line L5 (14.45, 61.22) -> (14.45, 48.42)
  line L6 (14.25, 48.42) -> (124.25, 48.42)
  point P0 (69.25, 50.42)
  dimension "d122" = 0.2
  constraints: 8 end point, 2 other
  measures "d122" distance between parallel lines of L1 L4
extrude "押し出し7" cut sketch "スケッチ9" against normal blind 13 contours L0 L1 L2 L6 L3 L4 L5
chamfer "面取り1" distance 1 angle 45 2 edges at (-54.8, 27, -10.8) (54.8, 27, -10.8)
equation "\"d3\" = d2"
equation "\"d46\" = d45"
equation "\"d86\" = d85"
equation "\"d87\" = 0.5 * d85"
equation "\"d95\" = 2 * d98"
equation "\"d105\" = 0.5 * d82"
